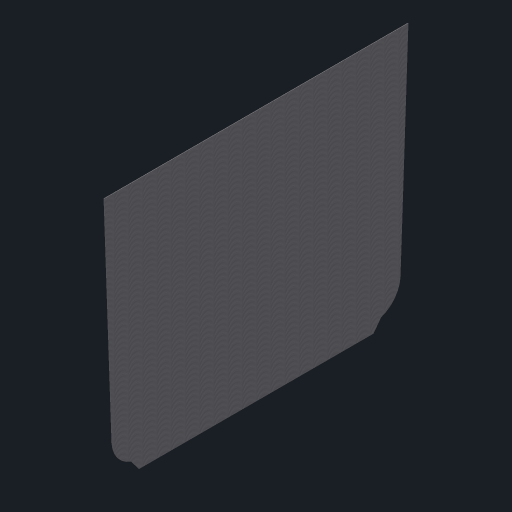
# Autodesk Inventor part: CHAPA_2
Saved by Autodesk Inventor 2024.3 (Build 283343000, 343)
## iProperties
Created: 2024-06-14
Part Number: CHAPA_2
Material: Steel, Mild, Welded
Document SubType Name: Sheet Metal
Designer: Niler
Density: 7.85 g/cm^3
Sheet Metal Rule: Default
Appearance: Weld - Steel Mild
Author: Niler
Autodesk Inventor part; units mm, degrees
ref_plane "YZ Plane" through (0, 0, 0) normal (1, 0, 0) x (0, 1, 0)
ref_plane "XZ Plane" through (0, 0, 0) normal (0, 1, 0) x (-1, 0, 0)
ref_plane "XY Plane" through (0, 0, 0) normal (0, 0, 1) x (1, 0, 0)
sketch "Sketch1" plane through (0, 0, 0) normal (1, 0, 0) x (0, 1, 0)
  line L0 (-41.95, 491.5) -> (41.95, 491.5)
  line L1 (41.95, 491.5) -> (41.95, -491.5)
  line L2 (41.95, -491.5) -> (-41.95, -491.5)
  line L3 (-41.95, -491.5) -> (-41.95, 491.5)
  line L4 (-41.95, 491.5) -> (41.95, -491.5) construction
  line L5 (41.95, 491.5) -> (-41.95, -491.5) construction
  line L6 (-41.95, 491.5) -> (-1012.9012, 456)
  line L7 (-1012.9012, 456) -> (-1012.9012, -456)
  line L8 (-1012.9012, -456) -> (-41.95, -491.5)
  line L9 (-332.05, 480.8933) -> (-332.05, -480.8933)
  line L10 (-1012.9012, 456) -> (-1126.9454, 370.3922)
  arc A0 (-1012.9012, 456) -> (-1094.1557, 395.0059) centre (-1009.649, 367.0481) ccw
  line L11 (-1012.9012, 0) -> (-1170.4564, 0)
  line L12 (-1126.9454, 370.3922) -> (-1126.9454, 0)
  line L13 (-1012.9012, -456) -> (-1126.9454, -370.3922)
  arc A1 (-1094.1557, -395.0059) -> (-1012.9012, -456) centre (-1009.649, -367.0481) ccw
  line L14 (-1126.9454, -370.3922) -> (-1126.9454, 0)
  point P0 (0, 0)
  point P1 (-41.95, 0)
  dimension "d0" = 983
  dimension "d1" = 83.9
  dimension "d3" = 912
  dimension "d4" = 971.6
  dimension "d5" = 374
  dimension "d9" = 34.8
  dimension "d10" = 101.6
  dimension "d11" = 41
  constraints: 30 end point, 5 point on line, 4 midpoint, 4 point on circle, 3 symmetric about line, 2 centre point, 2 horizontal, 2 parallel, 2 perpendicular, 2 vertical, 1 horizontal alignment, 1 tangent, 1 other
  measures "d0" distance of L0.end L1.end
  measures "d1" distance of L0.start L0.end
  measures "d3" distance of L6.end L7.end
  measures "d4" distance of L0.start L6.end
  measures "d5" distance between parallel lines of L9 L1
  measures "d9" angle of L6 L10
  measures "d10" distance of L6.end A0.end
  measures "d11" distance of L10.end A0.end
extrude "Plate2" add sketch "Sketch1" along normal blind 1.5 contours L9 L8 L7 L6
sheet face with bend "Face3" sketch "Sketch1" thickness 1.5 toward (1, 0, 0) bend radius 1.5 relief straight relief width 1.5 relief depth 0.75 contours L7 L11 L12 L10 | L10 A0 | L13 L14 L11 L7 | A1 L13
bend "Bend1"
equation "\"d7\" = Thickness"
equation "\"d12\" = BendRadius"
equation "\"d13\" = BendReliefWidth"
equation "\"d15\" = MinimumRemnant"
equation "\"d14\" = BendReliefDepth"
equation "\"d16\" = TransitionRadius"
equation "\"BendRadius\" = Thickness"
equation "\"BendReliefWidth\" = Thickness"
equation "\"BendReliefDepth\" = 0.5 * Thickness"
equation "\"CornerReliefSize\" = 4 * Thickness"
equation "\"MinimumRemnant\" = 2 * Thickness"
equation "\"TransitionRadius\" = BendRadius"
equation "\"JacobiRadiusSize\" = BendRadius"
equation "\"GapSize\" = Thickness"
equation "\"Thickness\" = 1.5"
body "Solid2"
